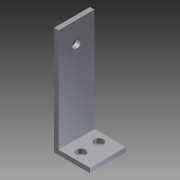
# Autodesk Inventor part: uptake support bracket
Saved by Autodesk Inventor 2012 (Build 160160000, 160)
## iProperties
Created: 2013-07-07
Part Number: uptake support bracket
Material: Default
Document SubType Name: Modeling
Designer: Bryce
Density: 1 g/cm^3
Author: Bryce
Autodesk Inventor part; units mm, degrees
ref_plane "YZ Plane" through (0, 0, 0) normal (1, 0, 0) x (0, 1, 0)
ref_plane "XZ Plane" through (0, 0, 0) normal (0, 1, 0) x (-1, 0, 0)
ref_plane "XY Plane" through (0, 0, 0) normal (0, 0, 1) x (1, 0, 0)
sketch "Sketch1" plane through (0, 0, 0) normal (0, 0, 1) x (1, 0, 0)
  line L0 (0, 0) -> (25.4, 0)
  line L1 (25.4, 0) -> (25.4, 3.175)
  line L2 (3.175, 76.2) -> (0, 76.2)
  line L3 (0, 76.2) -> (0, 0)
  line L4 (3.175, 76.2) -> (3.175, 3.175)
  line L5 (3.175, 3.175) -> (25.4, 3.175)
  dimension "d0" = 3.175
  dimension "d1" = 3.175
  dimension "d2" = 76.2
  dimension "d3" = 25.4
  constraints: 12 end point, 2 parallel, 1 horizontal, 1 perpendicular
  measures "d0" distance between parallel lines of L4 L3
  measures "d1" distance between parallel lines of L5 L0
  measures "d2" distance of L2.end L0.start
  measures "d3" distance of L0.start L0.end
extrude "Extrusion1" add sketch "Sketch1" along normal blind 25.4
sketch "Sketch2" plane through (0, 0, 0) normal (0, -1, 0) x (1, 0, 0)
  line L0 (25.4, 25.4) -> (0, 25.4) projected
  line L1 (0, 0) -> (25.4, 0) projected
  line L2 (25.4, 0) -> (25.4, 25.4) projected
  circle A0 centre (12.7, 19.05) radius 3.175
  circle A1 centre (12.7, 6.35) radius 3.175
  dimension "d17" = 25.4
  dimension "d6" = 12.7
  dimension "d7" = 6.35
  dimension "d8" = 6.35
  dimension "d9" = 6.35
  dimension "d10" = 6.35
  dimension "d11" = 12.7
  constraints: 2 centre point
  measures "d6" distance from line of L2 A0.centre
  measures "d7" distance from line of L0 A0.centre
  measures "d8" diameter of A0
  measures "d9" distance from line of L1 A1.centre
  measures "d10" diameter of A1
  measures "d11" distance from line of L2 A1.centre
extrude "Extrusion2" cut sketch "Sketch2" against normal blind 25.4
sketch "Sketch3" plane through (0, 0, 0) normal (-1, 0, 0) x (0, 0, 1)
  line L0 (25.4, 0) -> (25.4, 76.2) projected
  line L1 (0, 0) -> (25.4, 0) projected
  circle A0 centre (12.7, 61.7728) radius 3.175
  dimension "d14" = 6.35
  dimension "d15" = 61.7728
  dimension "d16" = 12.7
  constraints: 1 centre point
  measures "d14" diameter of A0
  measures "d15" distance from line of L1 A0.centre
  measures "d16" distance from line of L0 A0.centre
extrude "Extrusion3" cut sketch "Sketch3" against normal blind 25.4
equation "\"d1\" = d0"
equation "\"d10\" = d8"
equation "\"d11\" = d6"
body "Solid1"
